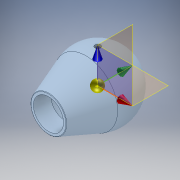
# Autodesk Inventor part: FilmLamp
Saved by Autodesk Inventor 2018.2 (Build 222227000, 227)
## iProperties
Created: 2018-01-26
Part Number: FilmLamp
Material: Beton
Document SubType Name: Modeling
Designer: JochenAlt
Density: 2.40731 g/cm^3
Appearance: Stahlblau - hell
Mass: 1482.18 g
Surface Area: 899.842 cm^2
Volume: 615.7 cm^3
Author: JochenAlt
Autodesk Inventor part; units mm, degrees
ref_plane "YZ Plane" through (0, 0, 0) normal (1, 0, 0) x (0, 1, 0)
ref_plane "XZ Plane" through (0, 0, 0) normal (0, 1, 0) x (-1, 0, 0)
ref_plane "XY Plane" through (0, 0, 0) normal (0, 0, 1) x (1, 0, 0)
sketch "Skizze1" plane through (0, 0, 0) normal (0, 0, 1) x (1, 0, 0)
  line L0 (0, 107.4807) -> (0, -123.0843) construction
  line L1 (-21.7268, 0) -> (95.361, 0) construction
  line L2 (6, 61.709) -> (6, 32.6387)
  line L3 (24.9064, -60.3552) -> (27.5, -90)
  line L4 (31.8067, -90) -> (27.5, -90)
  arc A0 (58.0619, -21.7443) -> (6, 61.709) centre (0, 0) ccw
  line L5 (58.0619, -21.7443) -> (32.7432, -89.3507)
  arc A1 (31.8067, -90) -> (32.7432, -89.3507) centre (31.8067, -89) ccw
  circle A2 centre (0, 0) radius 5
  arc A3 (24.9064, -60.3552) -> (6, 32.6387) centre (0, -17) ccw
  line L6 (52.4785, -36.6533) -> (46.8241, -34.5357) construction
  point P0 (32.5, -90)
  dimension "d3" = 6
  dimension "d11" = 62
  dimension "d12" = 5
  dimension "d13" = 90
  dimension "d15" = 5
  dimension "d16" = 27.5
  dimension "d17" = 1
  dimension "d18" = 10
  dimension "d68" = 100
  dimension "d69" = 17
  dimension "d70" = 6.0378
  constraints: 10 end point, 7 point on circle, 4 centre point, 4 point on line, 3 tangent, 2 coincident, 1 horizontal, 1 line through centre, 1 perpendicular, 1 vertical
  measures "d3" distance between parallel lines of L2 L0
  measures "d11" radius of A0
  measures "d12" angle of L0 L3
  measures "d13" distance between parallel lines of L1 L4
  measures "d15" distance of point (32.5, -90) L3.end
  measures "d16" distance from line of L0 L3.end
  measures "d17" radius of A1
  measures "d18" diameter of A2
  measures "d68" diameter of A3
  measures "d69" distance of A3.centre point (0, 0)
  measures "d70" distance of L6.end L6.start
revolve "Umdrehung1" add sketch "Skizze1" angle 360 about axis through (0, 0, 0) along (0, -1, 0) contours A0 L5 A1 L4 L3 A3 L2
extrude "Extrusion1" cut sketch "Skizze1" along normal through all both and the other way through all contours A2
sketch "Skizze3" plane through (0, 0, 0) normal (0, 0, 1) x (1, 0, 0)
  point P0 (0, 0)
